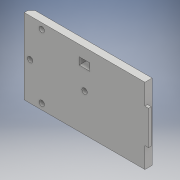
# Autodesk Inventor part: ttgorear
Saved by Autodesk Inventor 2017 (Build 210142000, 142)
## iProperties
Created: 2018-11-12
Part Number: ttgorear
Material: Generic
Document SubType Name: Modeling
Designer: simulator
Density: 1 g/cm^3
Appearance: Default
Author: simulator
## iProperties of the stored document ttgorear_3DPrint.ipt
Created: 2018-11-13
Part Number: ttgorear_3DPrint
Material: Generic
Document SubType Name: Modeling
Designer: simulator
Density: 1 g/cm^3
Appearance: Default
Author: simulator
Autodesk Inventor part; units mm, degrees
ref_plane "YZ Plane" through (0, 0, 0) normal (1, 0, 0) x (0, 1, 0)
ref_plane "XZ Plane" through (0, 0, 0) normal (0, 1, 0) x (-1, 0, 0)
ref_plane "XY Plane" through (0, 0, 0) normal (0, 0, 1) x (1, 0, 0)
sketch "Sketch1" plane through (0, 0, 0) normal (0, 1, 0) x (-1, 0, 0)
  arc A0 (67, -23) -> (69, -21) centre (67, -21) ccw
  line L0 (69, -21) -> (69, 21)
  arc A1 (69, 21) -> (67, 23) centre (67, 21) ccw
  line L1 (67, 23) -> (0, 23)
  arc A2 (0, 23) -> (-2, 21) centre (0, 21) ccw
  line L2 (-2, 21) -> (-2, -21)
  arc A3 (-2, -21) -> (0, -23) centre (0, -21) ccw
  line L3 (0, -23) -> (67, -23)
  line L4 (67, -21) -> (0, -21)
  line L5 (0, -21) -> (0, 21)
  line L6 (0, 21) -> (67, 21)
  line L7 (67, 21) -> (67, -21)
  line L8 (67, 21) -> (60.5, 21)
  line L9 (60.5, 21) -> (60.5, 14.5)
  line L10 (60.5, 14.5) -> (67, 14.5)
  line L11 (67, 14.5) -> (67, 21)
  line L12 (67, -21) -> (67, 21)
  line L13 (67, -21) -> (60.5, -21)
  line L14 (60.5, -21) -> (60.5, -14.5)
  line L15 (60.5, -14.5) -> (67, -14.5)
  line L16 (67, -14.5) -> (67, -21)
  line L17 (67, -21) -> (60.5, -14.5)
  line L18 (67, 21) -> (69, 21)
  line L19 (67, 21) -> (60.5, 14.5)
  line L20 (0, 16.25) -> (-2, 16.25)
  circle A4 centre (64.5, -18.5) radius 1
  circle A5 centre (64.5, 18.5) radius 1
  line L21 (60.5, -21) -> (0, -21)
  line L22 (0, -21) -> (0, 21)
  line L23 (0, 21) -> (60.5, 21)
  line L24 (60.5, 21) -> (60.5, 14.5)
  line L25 (60.5, 14.5) -> (67, 14.5)
  line L26 (67, 14.5) -> (67, -14.5)
  line L27 (67, -14.5) -> (60.5, -14.5)
  line L28 (60.5, -14.5) -> (60.5, -21)
  arc A6 (67, -23) -> (69, -21) centre (67, -21) ccw
  line L29 (69, -21) -> (69, 21)
  arc A7 (69, 21) -> (67, 23) centre (67, 21) ccw
  line L30 (67, 23) -> (0, 23)
  arc A8 (0, 23) -> (-2, 21) centre (0, 21) ccw
  line L31 (-2, 21) -> (-2, -21)
  arc A9 (-2, -21) -> (0, -23) centre (0, -21) ccw
  line L32 (0, -23) -> (67, -23)
  line L33 (-2, -10) -> (0, -10)
  line L34 (0, -10) -> (0, 10)
  line L35 (0, 10) -> (-2, 10)
  line L36 (-2, 10) -> (-2, -10)
  line L37 (0, -21) -> (4.5, -21)
  line L38 (67, 21) -> (0, 21)
  line L39 (0, 21) -> (0, -21)
  line L40 (0, -21) -> (67, -21)
  line L41 (67, -21) -> (67, 21)
  line L42 (0, 16.25) -> (-2, 16.25)
  line L43 (67, -21) -> (60.5, -21)
  line L44 (0, -21) -> (0, 21)
  line L45 (0, 21) -> (54, 21)
  line L46 (67, 21) -> (67, 3.25)
  arc A10 (67, -23) -> (69, -21) centre (67, -21) ccw
  line L47 (69, -21) -> (69, 21)
  arc A11 (69, 21) -> (67, 23) centre (67, 21) ccw
  line L48 (67, 23) -> (0, 23)
  arc A12 (0, 23) -> (-2, 21) centre (0, 21) ccw
  line L49 (-2, 21) -> (-2, -21)
  arc A13 (-2, -21) -> (0, -23) centre (0, -21) ccw
  line L50 (0, -23) -> (67, -23)
  line L51 (-2, -10) -> (0, -10)
  line L52 (0, -10) -> (0, 10)
  line L53 (0, 10) -> (-2, 10)
  line L54 (-2, 10) -> (-2, -10)
  line L55 (0, -21) -> (4.5, -21)
  line L56 (67, 21) -> (0, 21)
  line L57 (0, 21) -> (0, -21)
  line L58 (0, -21) -> (67, -21)
  line L59 (67, -21) -> (67, 21)
  line L60 (60.5, -21) -> (60.5, -14.5)
  line L61 (60.5, -14.5) -> (54, -14.5)
  line L62 (54, -14.5) -> (54, -21)
  line L63 (54, -21) -> (0, -21)
  line L64 (54, 21) -> (54, 14.5)
  line L65 (54, 14.5) -> (60.5, 14.5)
  line L66 (60.5, 14.5) -> (60.5, 21)
  line L67 (60.5, 21) -> (67, 21)
  line L68 (67, 3.25) -> (60.5, 3.25)
  line L69 (60.5, 3.25) -> (60.5, -3.25)
  line L70 (60.5, -3.25) -> (67, -3.25)
  line L71 (67, -3.25) -> (67, -21)
  line L72 (67, -3.25) -> (60.5, 3.25)
  line L73 (54, -14.5) -> (60.5, -21)
  line L74 (54, 14.5) -> (60.5, 21)
  point P0 (0, 0)
  point P1 (0, 0)
  point P2 (0, 0)
  point P3 (0, 0)
  point P4 (63.75, 0)
  point P5 (57.25, -17.75)
  point P6 (57.25, 17.75)
  dimension "d0" = 6.5
  dimension "d1" = 6.5
  dimension "d2" = 6.5
  dimension "d3" = 6.5
  dimension "d4" = 10
  dimension "d5" = 10
  dimension "d25" = 10
  dimension "d26" = 10
  constraints: 150 end point, 24 point on circle, 14 centre point, 13 parallel, 7 perpendicular, 6 horizontal, 5 point on line, 3 midpoint
  measures "d0" distance of L10.end L9.end
  measures "d1" distance of L9.end L8.end
  measures "d2" distance of L14.end L15.end
  measures "d3" distance of L13.end L14.end
  measures "d4" distance from line of point (0, 0) L35
  measures "d5" distance from line of point (0, 0) L33
  measures "d25" distance from line of point (0, 0) L53
  measures "d26" distance from line of point (0, 0) L51
extrude "Extrusion1" add sketch "Sketch1" along normal blind 2 contours L19 A5 L9 L6 | L7 L10 L19 A5 | L2 L35 L5 L33 | L74 L64 L6 | L9 L65 L74 | L7 L68 L69 L70 L15 L61 L62 L4 L5 L6 L64 L65 L10 | A5 L19 | L19 A5 | L7 L72 L68 | L70 L69 L72 | L7 L17 A4 L15 | L62 L73 L4 | L4 L14 L17 A4 | L14 L73 L61 | A4 L17 | L17 A4
sketch "Sketch2" plane through (0, 2, 0) normal (0, 1, 0) x (1, 0, 0)
  line L0 (0, -10) -> (2, -10) projected
  line L1 (2, -10) -> (2, 10) projected
  line L2 (2, 10) -> (0, 10) projected
  line L3 (0, 10) -> (0, 21) projected
  line L4 (0, 21) -> (-67, 21) projected
  line L5 (-67, 21) -> (-67, -21) projected
  line L6 (-67, -21) -> (0, -21) projected
  line L7 (0, -21) -> (0, -10) projected
  line L8 (-67, -21) -> (0, -21)
  line L9 (0, -21) -> (0, 21)
  line L10 (0, 21) -> (-67, 21)
  line L11 (-67, 21) -> (-67, -21)
  point P0 (0, 0)
  constraints: 8 end point, 2 parallel, 1 horizontal, 1 perpendicular
extrude "Extrusion2" add sketch "Sketch2" along normal blind 2 contours L7 L6 L5 L4 L3 L9
sketch "Sketch3" plane through (-67, 0, 21) normal (0, 0, 1) x (1, 0, 0)
  point P0 (67, 0)
sketch "Sketch4" plane through (0, 4, 0) normal (0, 1, 0) x (1, 0, 0)
  line L0 (0, 21) -> (-67, 21) projected
  line L1 (-67, 21) -> (-67, -21) projected
  line L2 (-67, -21) -> (0, -21) projected
  line L3 (0, -21) -> (0, 21) projected
  line L4 (0, 10) -> (0, 21) projected
  line L5 (0, 21) -> (-67, -21)
  point P0 (0, 0)
  point P1 (-33.5, 0)
  point P2 (-57.25, 17.75)
  point P3 (-63.75, 0)
  point P4 (-57.25, -17.75)
  point P5 (-57.25, 17.75)
  point P6 (-63.75, 0)
  point P7 (-57.25, -17.75)
  constraints: 3 coincident, 2 end point, 1 midpoint
hole "Hole1" at (-33.5, 4, 0) at (-57.25, 4, -17.75) at (-57.25, 4, 17.75) at (-63.75, 4, 0) direction (0, -1, 0) diameter 3 depth 8 tip angle 118
sketch "Sketch5" plane through (2, 0, 10) normal (1, 0, 0) x (0, 0, -1)
  line L0 (0, 0) -> (20, 0) projected
  line L1 (20, 0) -> (20, 2) projected
  line L2 (0, 2) -> (20, 2) projected
  line L3 (0, 0) -> (0, 2) projected
  line L4 (20, 2) -> (20, 0)
  line L5 (20, 0) -> (0, 0)
  line L6 (0, 0) -> (0, 2)
  line L7 (0, 2) -> (20, 2)
  line L8 (0, 0) -> (20, 0) projected
  line L9 (0.5, 0) -> (19.5, 0)
  line L10 (19.5, 0) -> (19.5, 1.5)
  line L11 (19.5, 1.5) -> (0.5, 1.5)
  line L12 (0.5, 1.5) -> (0.5, 0)
  point P0 (10, 0)
  dimension "d20" = 0.5
  dimension "d21" = 0.5
  dimension "d22" = 0.5
  constraints: 16 end point, 2 parallel, 2 point on line, 1 horizontal, 1 perpendicular, 3 other
  measures "d20" distance between parallel lines of L2 L11
  measures "d21" distance between parallel lines of L3 L12
  measures "d22" distance between parallel lines of L10 L1
extrude "Extrusion4" cut sketch "Sketch5" against normal up to surface (2 mm away) contours L3 L2 L1 L0 L10 L11 L12
sketch "Sketch6" plane through (0, 0, 0) normal (0, -1, 0) x (1, 0, 0)
  line L0 (-30.5, 15) -> (-36.5, 15)
  line L1 (-36.5, 15) -> (-36.5, 11)
  line L2 (-36.5, 11) -> (-30.5, 11)
  line L3 (-30.5, 11) -> (-30.5, 15)
  circle A0 centre (-63.75, 0) radius 1.5 projected
  circle A1 centre (-57.25, -17.75) radius 1.5 projected
  circle A2 centre (-33.5, 0) radius 1.5 projected
  circle A3 centre (-57.25, 17.75) radius 1.5 projected
  line L4 (2, 9.5) -> (0, 9.5) projected
  line L5 (0, 21) -> (0, 9.5) projected
  line L6 (-67, 21) -> (0, 21) projected
  line L7 (-67, -21) -> (-67, 21) projected
  line L8 (0, -21) -> (-67, -21) projected
  line L9 (0, -21) -> (0, -9.5) projected
  line L10 (0, -9.5) -> (2, -9.5) projected
  line L11 (2, 9.5) -> (2, -9.5) projected
  line L12 (-33.5, 21) -> (-33.5, 15)
  point P0 (0, 0)
  dimension "d27" = 4
  dimension "d28" = 6
  dimension "d29" = 6
  constraints: 10 end point, 2 midpoint, 2 parallel, 2 perpendicular, 1 horizontal
  measures "d27" distance of L0.end L1.end
  measures "d28" distance of L1.end L2.end
  measures "d29" distance of L12.end L12.start
extrude "Extrusion5" cut sketch "Sketch6" against normal through all contours L3 L2 L1 L0
chamfer "Chamfer1" distance 2 angle 45 1 edges at (-67, 4, 0)
body "Solid1"
